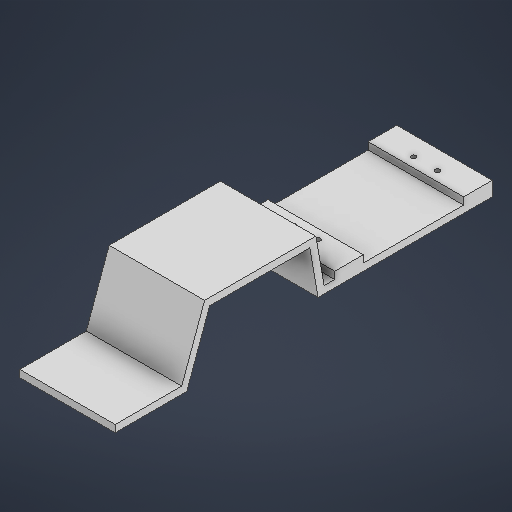
# Autodesk Inventor part: 1.2.4.UpperArmLink2
Saved by Autodesk Inventor 2026.1 (Build 301233020, 233B)
## iProperties
Created: 2025-10-08
Part Number: 1.2.4.UpperArmLink2
Material: Genérico
Document SubType Name: Modeling
Designer: vitos
Density: 1 g/cm^3
Appearance: Valor por defecto
Author: vitos
Autodesk Inventor part; units mm, degrees
ref_plane "YZ Plane" through (0, 0, 0) normal (1, 0, 0) x (0, 1, 0)
ref_plane "XZ Plane" through (0, 0, 0) normal (0, 1, 0) x (-1, 0, 0)
ref_plane "XY Plane" through (0, 0, 0) normal (0, 0, 1) x (1, 0, 0)
sketch "Boceto1" plane through (0, 0, 0) normal (1, 0, 0) x (0, 1, 0)
  line L0 (3, 30) -> (0, 30)
  line L1 (0, 30) -> (0, 0)
  line L2 (0, 0) -> (26.3114, -9.5766)
  line L3 (0, 0) -> (28, 0) construction
  line L4 (26.3114, -9.5766) -> (26.3114, -51.5766)
  line L5 (26.3114, -51.5766) -> (6.6152, -55.0495)
  line L6 (6.6152, -55.0495) -> (6.6152, -128.0495)
  line L7 (6.6152, -128.0495) -> (9.6152, -128.0495)
  line L8 (9.6152, -128.0495) -> (9.6152, -57.5668)
  line L9 (6.6152, -55.0495) -> (6.6152, -58.0495)
  line L10 (29.3114, -9.5766) -> (29.3114, -54.0939)
  line L11 (27.3375, -6.7575) -> (3, 2.1006)
  line L12 (3, 2.1006) -> (3, 30)
  line L13 (29.3114, -54.0939) -> (9.6152, -57.5668)
  line L14 (27.3375, -6.7575) -> (29.3114, -7.4759)
  line L15 (29.3114, -9.5766) -> (29.3114, -7.4759)
  dimension "d0" = 3
  dimension "d2" = 28
  dimension "d3" = 20
  dimension "d6" = 100
  dimension "d7" = 73
  dimension "d8" = 3
  dimension "d9" = 3
  dimension "d12" = 3
  dimension "d13" = 3
  constraints: 32 end point, 2 parallel, 2 perpendicular, 2 vertical, 1 collinear, 1 equal length, 1 horizontal, 1 point on line
  measures "d0" distance of L0.end L0.start
  measures "d2" distance of L1.end L2.end
  measures "d3" angle of L2 L3
  measures "d6" angle of L4 L5
  measures "d7" distance of L5.end L6.end
  measures "d8" distance of L6.end L7.end
  measures "d9" distance of L5.end L9.end
  measures "d12" distance of L2.end L11.start
  measures "d13" distance of L2.end L10.start
extrude "Extrusión1" add sketch "Boceto1" along normal blind 40
sketch "Boceto4" plane through (0, 9.6152, -57.5668) normal (0, 1, 0) x (1, 0, 0)
  line L0 (0, 70.4827) -> (40, 70.4827) projected
  line L1 (40, -2.5173) -> (40, 70.4827) projected
  line L2 (0, 70.4827) -> (40, 70.4827)
  line L3 (40, 70.4827) -> (40, 58.4827)
  line L4 (40, 58.4827) -> (0, 58.4827)
  line L5 (0, 58.4827) -> (0, 70.4827)
  line L6 (11, 58.4827) -> (30, 58.4827)
  line L7 (30, 58.4827) -> (30, 16.4827)
  line L8 (30, 16.4827) -> (11, 16.4827)
  line L9 (11, 16.4827) -> (11, 58.4827)
  line L10 (0, 16.4827) -> (40, 16.4827)
  line L11 (40, 16.4827) -> (40, 4.4827)
  line L12 (40, 4.4827) -> (0, 4.4827)
  line L13 (0, 4.4827) -> (0, 16.4827)
  circle A0 centre (25, 62.483) radius 1
  circle A1 centre (15, 62.483) radius 1
  circle A2 centre (25, 12.483) radius 1
  circle A3 centre (15, 12.483) radius 1
  point P0 (0, -57.5668)
  point P1 (30, 16.4827)
  dimension "d22" = 12
  dimension "d23" = 19
  dimension "d24" = 42
  dimension "d25" = 12
  dimension "d26" = 2
  dimension "d27" = 2
  dimension "d28" = 2
  dimension "d29" = 2
  constraints: 24 end point, 6 parallel, 5 point on line, 4 centre point, 3 horizontal, 3 perpendicular
  measures "d22" distance of L2.end L3.end
  measures "d23" distance of L7.end L8.end
  measures "d24" distance of L6.end L7.end
  measures "d25" distance of L10.end L11.end
  measures "d26" diameter of A0
  measures "d27" diameter of A1
  measures "d28" diameter of A2
  measures "d29" diameter of A3
extrude "Extrusión4" add sketch "Boceto4" along normal blind 3 contours L0 L1 L4 L5 | L1 L12 L13 L10 L8
extrude "Extrusión5" cut sketch "Boceto4" against normal blind 3 contours A0 | A1 | A2 | A3
thread "Rosca1" size "M2x0.4" class "6H" standard "ANSI Metric M Profile" full length
thread "Rosca2" size "M2x0.4" class "6H" standard "ANSI Metric M Profile" full length
thread "Rosca3" size "M2x0.4" class "6H" standard "ANSI Metric M Profile" full length
thread "Rosca4" size "M2x0.4" class "6H" standard "ANSI Metric M Profile" full length
